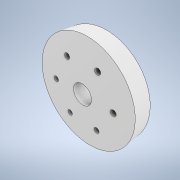
# Autodesk Inventor part: Spool Hub
Saved by Autodesk Inventor 2020 (Build 240168000, 168)
## iProperties
Created: 2020-02-04
Part Number: Spool Hub
Material: Acetal Resin, White
Document SubType Name: Modeling
Designer: JimAndVal
Density: 1.425 g/cm^3
Appearance: Smooth - White
Author: JimAndVal
Autodesk Inventor part; units mm, degrees
ref_plane "YZ Plane" through (0, 0, 0) normal (1, 0, 0) x (0, 1, 0)
ref_plane "XZ Plane" through (0, 0, 0) normal (0, 1, 0) x (-1, 0, 0)
ref_plane "XY Plane" through (0, 0, 0) normal (0, 0, 1) x (1, 0, 0)
sketch "Sketch1" plane through (0, 0, 0) normal (0, 0, 1) x (1, 0, 0)
  circle A0 centre (23.8125, 0) radius 2.1463
  circle A1 centre (11.9063, 20.6222) radius 2.1463
  circle A2 centre (-11.9062, 20.6222) radius 2.1463
  circle A3 centre (-23.8125, 0) radius 2.1463
  circle A4 centre (-11.9063, -20.6222) radius 2.1463
  circle A5 centre (11.9062, -20.6222) radius 2.1463
  circle A6 centre (0, 0) radius 38.1
  circle A7 centre (0, 0) radius 7.62
  dimension "d0" = 4.2926
  dimension "d4" = 360
  dimension "d6" = 76.2
  dimension "d9" = 15.24
  constraints: 8 centre point, 2 coincident, 13 other
  measures "d0" diameter of A0
  measures "d6" diameter of A6
  measures "d9" diameter of A7
extrude "Extrusion1" add sketch "Sketch1" along normal mid plane 12.7
body "Solid1"
